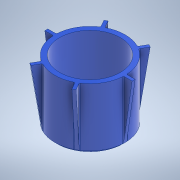
# Autodesk Inventor part: tail
Saved by Autodesk Inventor 2020 (Build 240168000, 168)
## iProperties
Created: 2021-01-23
Part Number: tail
Material: ABS Plastic
Document SubType Name: Modeling
Designer: 0x6f736f646f
Density: 1.06 g/cm^3
Appearance: Smooth - White
Author: 0x6f736f646f
Autodesk Inventor part; units mm, degrees
ref_plane "YZ Plane" through (0, 0, 0) normal (1, 0, 0) x (0, 1, 0)
ref_plane "XZ Plane" through (0, 0, 0) normal (0, 1, 0) x (-1, 0, 0)
ref_plane "XY Plane" through (0, 0, 0) normal (0, 0, 1) x (1, 0, 0)
sketch "Sketch1" plane through (0, 0, 0) normal (0, 1, 0) x (-1, 0, 0)
  circle A0 centre (0, 0) radius 50
  circle A1 centre (0, 0) radius 54
  circle A2 centre (0, 0) radius 58
  dimension "d0" = 100
  dimension "d1" = 108
  dimension "d2" = 116
  constraints: 3 centre point, 3 coincident
  measures "d0" diameter of A0
  measures "d1" diameter of A1
  measures "d2" diameter of A2
extrude "Extrusion1" add sketch "Sketch1" along normal blind 96 and the other way blind 4 contours A1
extrude "Extrusion2" add sketch "Sketch1" along normal blind 96 contours A2
sketch "Sketch3" plane through (0, 0, 0) normal (0, 0, 1) x (1, 0, 0)
  line L0 (-54, 0) -> (54, 0) projected
  line L1 (-54, 0) -> (-54, 96)
  line L2 (58, 96) -> (-58, 96) projected
  line L3 (-54, 96) -> (-72, 96)
  line L4 (-72, 96) -> (-58, 0)
  line L5 (-58, 0) -> (-58, 96) projected
  line L6 (58, 0) -> (-58, 0) projected
  line L7 (-58, 0) -> (-54, 0)
  point P0 (0, 0)
  dimension "d10" = 18
  constraints: 8 end point, 2 point on line, 1 collinear, 1 horizontal, 1 vertical
  measures "d10" distance of L1.end L3.end
extrude "Extrusion3" add sketch "Sketch3" along normal mid plane 5
fillet "Fillet1" radius 2 2 edges at (-57.9461, 48, 2.5) (-57.9461, 48, -2.5)
pattern_circular "Circular Pattern1" count 6 over 360 about axis through (0, -10, 0) along (0, 1, 0) of "Extrusion3", "Fillet1"
body "Solid1"
